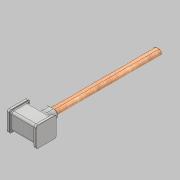
# Autodesk Inventor part: exercise3-9-10
Saved by Autodesk Inventor 2018 (Build 220112000, 112)
## iProperties
Created: 2020-09-23
Part Number: exercise3-9-10
Material: 一般
Document SubType Name: Modeling
Designer: 王鼎鈞
Density: 1 g/cm^3
Appearance: 預設
Author: 王鼎鈞
Autodesk Inventor part; units mm, degrees
ref_plane "YZ Plane" through (0, 0, 0) normal (1, 0, 0) x (0, 1, 0)
ref_plane "XZ Plane" through (0, 0, 0) normal (0, 1, 0) x (-1, 0, 0)
ref_plane "XY Plane" through (0, 0, 0) normal (0, 0, 1) x (1, 0, 0)
sketch "草圖1" plane through (0, 0, 0) normal (1, 0, 0) x (0, 1, 0)
  line L0 (-50, 50) -> (50, 50)
  line L1 (50, 50) -> (50, -50)
  line L2 (50, -50) -> (-50, -50)
  line L3 (-50, -50) -> (-50, 50)
  line L4 (-50, 50) -> (50, -50) construction
  line L5 (50, 50) -> (-50, -50) construction
  point P0 (0, 0)
  point P1 (0, 0)
  dimension "d0" = 100
  dimension "d1" = 100
  constraints: 12 end point, 2 midpoint, 2 parallel, 1 horizontal, 1 perpendicular
  measures "d0" distance of L1.end L2.end
  measures "d1" distance of L2.end L0.start
extrude "擠出1" add sketch "草圖1" along normal blind 12
fillet "圓角1" radius 10 4 edges at (6, 50, 50) (6, -50, 50) (6, -50, -50) (6, 50, -50)
chamfer "倒角1" distance 1 angle 45 16 edges at (12, 0, 50) (12, -47.0711, 47.0711) (12, -50, 0) (12, -47.0711, -47.0711) (12, 0, -50) (12, 47.0711, -47.0711) (12, 50, 0) (12, 47.0711, 47.0711) (0, 0, 50) (0, 47.0711, 47.0711) (0, 50, 0) (0, 47.0711, -47.0711) (0, 0, -50) (0, -47.0711, -47.0711) (0, -50, 0) (0, -47.0711, 47.0711)
sketch "草圖2" plane through (12, 0, 0) normal (1, 0, 0) x (0, 0, -1)
  line L0 (-30, -30) -> (30, -30)
  line L1 (30, -30) -> (30, 30)
  line L2 (30, 30) -> (-30, 30)
  line L3 (-30, 30) -> (-30, -30)
  line L4 (-30, -30) -> (30, 30) construction
  line L5 (30, -30) -> (-30, 30) construction
  line L6 (-30, 30) -> (30, 30)
  line L7 (30, 30) -> (30, 42)
  line L8 (30, 42) -> (-30, 42)
  line L9 (-30, 42) -> (-30, 30)
  line L10 (-30, 30) -> (-42, 30)
  line L11 (-42, 30) -> (-42, -30)
  line L12 (-42, -30) -> (-30, -30)
  line L13 (-30, -30) -> (-30, 30)
  line L14 (-30, -30) -> (30, -30)
  line L15 (30, -30) -> (30, -42)
  line L16 (30, -42) -> (-30, -42)
  line L17 (-30, -42) -> (-30, -30)
  line L18 (30, 30) -> (42, 30)
  line L19 (42, 30) -> (42, -30)
  line L20 (42, -30) -> (30, -30)
  line L21 (30, -30) -> (30, 30)
  point P0 (0, 0)
  dimension "d8" = 60
  dimension "d9" = 60
  dimension "d10" = 12
  dimension "d11" = 12
  dimension "d12" = 12
  dimension "d13" = 12
  constraints: 44 end point, 10 parallel, 5 horizontal, 5 perpendicular, 2 midpoint, 1 point on line
  measures "d8" distance of L2.end L1.end
  measures "d9" distance of L1.end L0.end
  measures "d10" distance of L7.end L6.end
  measures "d11" distance of L12.end L11.end
  measures "d12" distance of L14.end L15.end
  measures "d13" distance of L19.end L20.end
extrude "擠出2" add sketch "草圖2" along normal blind 120 contours L12 L11 L10 L3 | L0 L15 L16 L17 | L1 L18 L19 L20 | L9 L8 L7 L2
sketch "草圖3" plane through (132, 0, 0) normal (1, 0, 0) x (0, 0, -1)
  arc A0 (-40, 50) -> (-50, 40) centre (-40, 40) ccw projected
  line L0 (-50, 40) -> (-50, -40) projected
  line L1 (40, 50) -> (-40, 50) projected
  arc A1 (-50, -40) -> (-40, -50) centre (-40, -40) ccw projected
  line L2 (-40, -50) -> (40, -50) projected
  arc A2 (40, -50) -> (50, -40) centre (40, -40) ccw projected
  line L3 (50, -40) -> (50, 40) projected
  arc A3 (50, 40) -> (40, 50) centre (40, 40) ccw projected
  point P0 (0, 0)
extrude "擠出3" add sketch "草圖3" along normal blind 12
chamfer "倒角2" distance 1 angle 45 16 edges at (144, -47.0711, -47.0711) (144, 0, -50) (144, 47.0711, -47.0711) (144, 50, 0) (144, 47.0711, 47.0711) (144, 0, 50) (144, -47.0711, 47.0711) (144, -50, 0) (132, -50, 0) (132, -47.0711, -47.0711) (132, 0, -50) (132, 47.0711, -47.0711) (132, 50, 0) (132, 47.0711, 47.0711) (132, 0, 50) (132, -47.0711, 47.0711)
delete faces "刪除面1" heal yes whole lump no faces at (92, -30, 38) (92, -34, 30)
delete faces "刪除面2" heal yes whole lump no faces at (92, -38, -30) (92, -30, -34) (92, 30, -38) (92, 34, -30) (92, 30, 34) (92, 38, 30)
fillet "圓角2" radius 10 4 edges at (72, -42, -42) (72, 42, 42) (72, 42, -42) (72, -42, 42)
fillet "圓角3" radius 4 16 edges at (12, 42, 0) (12, 39.0711, 39.0711) (12, 0, 42) (12, -39.0711, 39.0711) (12, -42, 0) (12, -39.0711, -39.0711) (12, 0, -42) (12, 39.0711, -39.0711) (132, 0, -42) (132, -39.0711, -39.0711) (132, -42, 0) (132, -39.0711, 39.0711) (132, 0, 42) (132, 39.0711, 39.0711) (132, 42, 0) (132, 39.0711, -39.0711)
sketch "草圖4" plane through (16, 42, -32) normal (0, 1, 0) x (1, 0, 0)
  arc A0 (116, -78) -> (112, -74) centre (112, -78) ccw projected
  line L0 (0, -64) -> (0, -74) projected
  line L1 (-44.8, -32) -> (156.8, -32) projected
  line L2 (-16, 45.0469) -> (-16, -103.1745) projected
  line L3 (-4, -72) -> (-4, -81) projected
  line L4 (56, -72) -> (56, -81)
  line L5 (56, -72) -> (56, 23.8724)
  line L6 (26, -52) -> (86, -52)
  line L7 (86, -52) -> (86, -12)
  line L8 (86, -12) -> (26, -12)
  line L9 (26, -12) -> (26, -52)
  line L10 (26, -52) -> (86, -12) construction
  line L11 (86, -52) -> (26, -12) construction
  line L12 (36, -19.5) -> (76, -19.5)
  line L13 (76, -19.5) -> (76, -44.5)
  line L14 (76, -44.5) -> (36, -44.5)
  line L15 (36, -44.5) -> (36, -19.5)
  line L16 (36, -19.5) -> (76, -44.5) construction
  line L17 (76, -19.5) -> (36, -44.5) construction
  point P0 (-16, -32)
  point P1 (56, -32)
  point P2 (56, -32)
  dimension "d23" = 60
  dimension "d24" = 60
  dimension "d25" = 40
  dimension "d26" = 40
  dimension "d27" = 25
  constraints: 28 end point, 6 midpoint, 5 parallel, 2 horizontal, 2 perpendicular, 1 point on line, 1 vertical
  measures "d23" distance between parallel lines of L3 L4
  measures "d24" distance of L8.end L7.end
  measures "d25" distance of L7.end L6.end
  measures "d26" distance of L13.end L14.end
  measures "d27" distance of L12.end L13.end
extrude "擠出4" add sketch "草圖4" along normal blind 60 contours L9 L8 L5 L12 L15 L1 | L1 L15 L14 L5 L6 L9 | L8 L7 L1 L13 L12 L5 | L5 L14 L13 L1 L7 L6
fillet "圓角4" radius 20 4 edges at (42, 72, -20) (42, 72, 20) (102, 72, -20) (102, 72, 20)
fillet "圓角5" radius 12.5 4 edges at (92, 72, -12.5) (92, 72, 12.5) (52, 72, -12.5) (52, 72, 12.5)
fillet "圓角6" radius 3 8 edges at (72, 42, -20) (42, 42, 0) (47.8578, 42, -14.1422) (47.8578, 42, 14.1422) (72, 42, 20) (96.1422, 42, -14.1422) (96.1422, 42, 14.1422) (102, 42, 0)
chamfer "倒角3" distance 5 angle 45 8 edges at (42, 102, 0) (47.8578, 102, -14.1422) (47.8578, 102, 14.1422) (72, 102, -20) (96.1422, 102, -14.1422) (96.1422, 102, 14.1422) (102, 102, 0) (72, 102, 20)
sketch "草圖5" plane through (64.5, 42, 12.5) normal (0, 1, 0) x (1, 0, 0)
  arc A0 (0, 25) -> (0, 0) centre (0, 12.5) ccw projected
  line L0 (0, 0) -> (15, 0) projected
  arc A1 (15, 0) -> (15, 25) centre (15, 12.5) ccw projected
  line L1 (15, 25) -> (0, 25) projected
  point P0 (-64.5, 12.5)
extrude "擠出5" add sketch "草圖5" along normal blind 583.75
fillet "圓角7" radius 5 4 edges at (72, 625.75, -12.5) (52, 625.75, 0) (72, 625.75, 12.5) (92, 625.75, 0)
